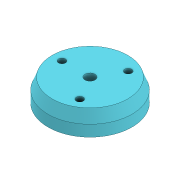
# Autodesk Inventor part: bevel-gear-side
Saved by Autodesk Inventor 2020.3 (Build 243373000, 373)
## iProperties
Created: 2021-06-13
Part Number: bevel-gear-side
Material: Generic
Document SubType Name: Modeling
Designer: Yusuf
Mass: 5.18231 g
Surface Area: 22.6806 cm^2
Volume: 5.18231 cm^3
Density: 1 g/cm^3
Appearance: Cadet Blue
Author: Yusuf
Autodesk Inventor part; units mm, degrees
ref_plane "YZ Plane" through (0, 0, 0) normal (1, 0, 0) x (0, 1, 0)
ref_plane "XZ Plane" through (0, 0, 0) normal (0, 1, 0) x (-1, 0, 0)
ref_plane "XY Plane" through (0, 0, 0) normal (0, 0, 1) x (1, 0, 0)
sketch "Sketch1" plane through (0, 0, 0) normal (0, 1, 0) x (-1, 0, 0)
  circle A0 centre (-5, -8.6603) radius 1.25
  circle A1 centre (-5, -8.6603) radius 1
  circle A2 centre (10, 0) radius 1
  circle A3 centre (10, 0) radius 1
  circle A4 centre (-5, 8.6603) radius 1
  circle A5 centre (-5, 8.6603) radius 1
  circle A6 centre (0, 0) radius 1.8
  circle A7 centre (0, 0) radius 15
  circle A8 centre (10, 0) radius 1.25
  circle A9 centre (-5, 8.6603) radius 1.25
  dimension "d1" = 3.6
  dimension "d2" = 30
  dimension "d3" = 8.6602
  dimension "d4" = 10
  dimension "d5" = 10
  dimension "d6" = 10
  dimension "d7" = 2.5
  dimension "d8" = 2.5
  dimension "d9" = 2.5
  constraints: 10 centre point, 7 coincident, 1 horizontal alignment, 1 vertical alignment
  measures "d1" diameter of A6
  measures "d2" diameter of A7
  measures "d3" vertical distance of A1.centre A6.centre
  measures "d4" distance of A1.centre A6.centre
  measures "d5" distance of A5.centre A6.centre
  measures "d6" distance of A3.centre A6.centre
  measures "d7" diameter of A0
  measures "d8" diameter of A8
  measures "d9" diameter of A9
extrude "Extrusion1" add sketch "Sketch1" along normal blind 8 contours A7
chamfer "Chamfer1" distance 1.5 distance2 4 1 edges at (15, 8, 0) measured on face at (-6.2778, 8, -4.9516)
body "Solid1"
